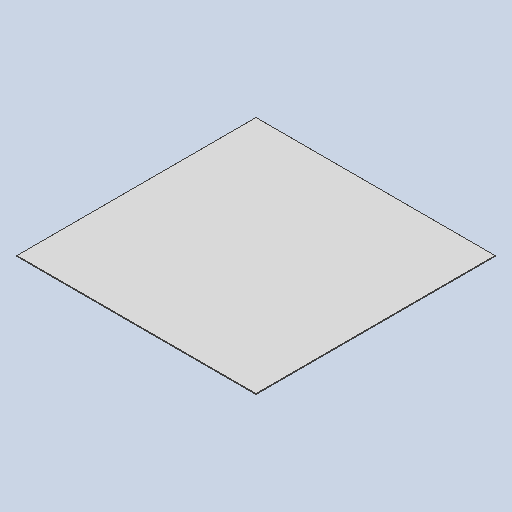
# Autodesk Inventor part: 0931_CPY1
Saved by Autodesk Inventor 2026 (Build 300175000, 175)
## iProperties
Created: 2026-05-19
Part Number: 0931_CPY1
Material: Типовые
Document SubType Name: Sheet Metal
Designer: user
Density: 1 g/cm^3
Sheet Metal Rule: По умолчанию_мм
Appearance: По умолчанию
Author: user
Autodesk Inventor part; units mm, degrees
ref_plane "YZ Plane" through (0, 0, 0) normal (1, 0, 0) x (0, 1, 0)
ref_plane "XZ Plane" through (0, 0, 0) normal (0, 1, 0) x (-1, 0, 0)
ref_plane "XY Plane" through (0, 0, 0) normal (0, 0, 1) x (1, 0, 0)
sketch "Эскиз1" plane through (0, 0, 0) normal (0, 1, 0) x (-1, 0, 0)
  line L0 (750, 750) -> (-750, 750)
  line L1 (-750, 750) -> (-750, -750)
  line L2 (-750, -750) -> (750, -750)
  line L3 (750, -750) -> (750, 750)
  line L4 (750, 750) -> (-750, -750) construction
  line L5 (-750, 750) -> (750, -750) construction
  point P0 (0, 0)
  dimension "d0" = 1500
  dimension "d1" = 1500
  measures "d0" distance of L2.end L1.end
  measures "d1" distance of L1.end L0.end
extrude "Пластина1" add sketch "Эскиз1" along normal blind 5
equation "\"d2\" = Толщина"
equation "\"Радиус_гибки\" = Толщина"
equation "\"Ширина_просечки\" = Толщина"
equation "\"Глубина_просечки\" = 0.5 * Толщина"
equation "\"Радиус_перехода\" = Радиус_гибки"
equation "\"Радиус_Якоби\" = Радиус_гибки"
equation "\"Размер_зазора\" = Толщина"
equation "\"Толщина\" = 5"
